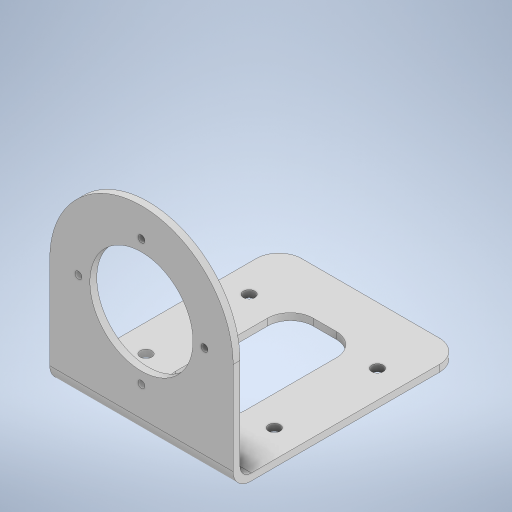
# Autodesk Inventor part: Holder Water Pump
Saved by Autodesk Inventor 2024 (Build 280153000, 153)
## iProperties
Created: 2024-06-17
Part Number: Holder Water Pump
Material: Generic
Document SubType Name: Modeling
Designer: ASUS
Density: 1 g/cm^3
Appearance: Default
Author: ASUS
Autodesk Inventor part; units mm, degrees
ref_plane "YZ Plane" through (0, 0, 0) normal (1, 0, 0) x (0, 1, 0)
ref_plane "XZ Plane" through (0, 0, 0) normal (0, 1, 0) x (-1, 0, 0)
ref_plane "XY Plane" through (0, 0, 0) normal (0, 0, 1) x (1, 0, 0)
sketch "Sketch1" plane through (0, 0, 0) normal (0, 1, 0) x (-1, 0, 0)
  line L0 (40, 50) -> (-40, 50)
  line L1 (-40, 50) -> (-40, -50)
  line L2 (-40, -50) -> (40, -50)
  line L3 (40, -50) -> (40, 50)
  line L4 (40, 50) -> (-40, -50) construction
  line L5 (-40, 50) -> (40, -50) construction
  point P0 (0, 0)
  dimension "d0" = 80
  dimension "d1" = 100
  constraints: 12 end point, 2 midpoint, 2 parallel, 1 horizontal, 1 perpendicular
  measures "d0" distance of L1.end L2.end
  measures "d1" distance of L2.end L0.start
extrude "Extrusion1" add sketch "Sketch1" along normal blind 3
sketch "Sketch2" plane through (0, 3, 0) normal (0, 1, 0) x (1, 0, 0)
  line L0 (-40, 50) -> (-40, -50) projected
  line L1 (40, -50) -> (40, 50) projected
  line L2 (-40, -50) -> (40, -50)
  line L3 (40, -50) -> (40, -47)
  line L4 (40, -47) -> (-40, -47)
  line L5 (-40, -47) -> (-40, -50)
  point P0 (0, 0)
  dimension "d4" = 3
  constraints: 8 end point, 2 parallel, 1 horizontal, 1 perpendicular, 1 point on line
  measures "d4" distance of L1.start L3.end
extrude "Extrusion2" add sketch "Sketch2" along normal blind 85
sketch "Sketch4" plane through (40, 3, 47) normal (0, 0, -1) x (-1, 0, 0)
  circle A0 centre (40, 45) radius 22.5
  line L0 (0, 0) -> (80, 0) projected
  line L1 (0, 0) -> (0, 85) projected
  circle A1 centre (12.5, 45) radius 1.5
  circle A2 centre (40, 72.5) radius 1.5
  circle A3 centre (67.5, 45) radius 1.5
  circle A4 centre (40, 17.5) radius 1.5
  line L2 (0, 85) -> (80, 85) projected
  point P0 (40, -3)
  dimension "d7" = 45
  dimension "d9" = 40
  dimension "d10" = 3
  dimension "d11" = 3
  dimension "d12" = 3
  dimension "d13" = 3
  dimension "d14" = 27.5
  dimension "d15" = 27.5
  dimension "d16" = 27.5
  dimension "d17" = 27.5
  dimension "d21" = 40
  constraints: 5 centre point, 2 horizontal alignment, 2 vertical alignment
  measures "d7" diameter of A0
  measures "d9" distance from line of L1 A0.centre
  measures "d10" diameter of A1
  measures "d11" diameter of A4
  measures "d12" diameter of A3
  measures "d13" diameter of A2
  measures "d14" distance of A3.centre A0.centre
  measures "d15" distance of A2.centre A0.centre
  measures "d16" distance of A0.centre A4.centre
  measures "d17" distance of A1.centre A0.centre
  measures "d21" distance from line of L2 A0.centre
extrude "Extrusion3" cut sketch "Sketch4" against normal blind 3
fillet "Fillet1" radius 40 2 edges at (40, 88, 48.5) (-40, 88, 48.5)
fillet "Fillet2" radius 5 1 edges at (0, 3, 47)
fillet "Fillet3" radius 7.5 1 edges at (0, 0, 50)
fillet "Fillet4" radius 10 2 edges at (40, 1.5, -50) (-40, 1.5, -50)
sketch "Sketch7" plane through (0, 3, 0) normal (0, 1, 0) x (1, 0, 0)
  circle A0 centre (28, -20) radius 2.5
  circle A1 centre (28, 25) radius 2.5
  circle A2 centre (-28, 25) radius 2.5
  circle A3 centre (-28, -20) radius 2.5
  line L0 (40, -42) -> (40, 40) projected
  line L1 (30, 50) -> (-30, 50) projected
  line L2 (-40, 40) -> (-40, -42) projected
  line L3 (15, -30) -> (-15, -30)
  line L4 (-15, -30) -> (-15, 30)
  line L5 (-15, 30) -> (15, 30)
  line L6 (15, 30) -> (15, -30)
  line L7 (15, -30) -> (-15, 30) construction
  line L8 (-15, -30) -> (15, 30) construction
  point P0 (0, 0)
  dimension "d25" = 5
  dimension "d26" = 5
  dimension "d27" = 5
  dimension "d28" = 5
  dimension "d29" = 12
  dimension "d30" = 70
  dimension "d31" = 25
  dimension "d32" = 12
  dimension "d33" = 70
  dimension "d34" = 25
  dimension "d35" = 30
  dimension "d36" = 60
  constraints: 12 end point, 4 centre point, 2 midpoint, 2 parallel, 2 vertical alignment, 1 horizontal, 1 perpendicular
  measures "d25" diameter of A0
  measures "d26" diameter of A3
  measures "d27" diameter of A2
  measures "d28" diameter of A1
  measures "d29" distance from line of L0 A0.centre
  measures "d30" distance from line of A0.centre L1
  measures "d31" distance from line of L1 A1.centre
  measures "d32" distance from line of L2 A3.centre
  measures "d33" distance from line of L1 A3.centre
  measures "d34" distance from line of L1 A2.centre
  measures "d35" distance between parallel lines of L4 L6
  measures "d36" distance of L3.end L4.end
extrude "Extrusion4" cut sketch "Sketch7" against normal blind 85
fillet "Fillet5" radius 10 4 edges at (-15, 1.5, 30) (15, 1.5, 30) (15, 1.5, -30) (-15, 1.5, -30)
body "Solid1"
